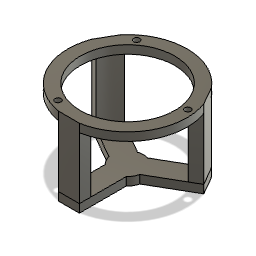
Speaker Mount Parts (Autodesk Fusion 360 design; units mm, degrees)
Autodesk Fusion 360 part; units mm, degrees
note: some values were not read from the file. Set by a fixed rule: which sketch regions a step uses; the direction of a hole.
sketch "Sketch1" plane through (0, 0, 0) normal (0, 1, 0) x (1, 0, 0)
  circle A0 centre (0, 0) radius 25.75
  line L0 (0, 0) -> (0, -25.75) construction
  line L1 (0, -30.75) -> (0, -25.75) construction
  line L2 (5.7222, -25.75) -> (-5.7222, -25.75)
  line L3 (-5.7222, -25.75) -> (-5.7222, -31.9923)
  line L4 (-5.7222, -31.9923) -> (5.7222, -31.9923)
  line L5 (5.7222, -31.9923) -> (5.7222, -25.75)
  circle A1 centre (0, 0) radius 32.5
  dimension "d1" = 51.5
  dimension "d62" = 11.4444
  dimension "d83" = 65
  constraint coincident A0.centre L0.start
  constraint coincident A0 L0.end
  constraint vertical L0
  constraint perpendicular L2 L3
  constraint parallel L2 L4
  constraint parallel L3 L5
  constraint perpendicular L1 L2
  constraint midpoint L0.end L2
  constraint concentric A0 A1
  constraint coincident L4.end A1
  constraint horizontal L2
  measures "d1" diameter of A0
  measures "d62" distance of L3.end L4.end
  measures "d83" diameter of A1
extrude "Extrude1" add sketch "Sketch1" along normal mid plane 4.5 makes body 1
extrude "Extrude6" cut sketch "Sketch1" along normal up to surface (2.25 mm away) and the other way up to surface (2.25 mm away) contours L4 A1 bodies 1
pattern_circular "C-Pattern2" count 3 over 360 about axis through (0, 1.75, 0) along (0, 1, 0) of "Extrude6"
ref_plane "WorkPlane1" through (0, 2.25, 0) normal (0, 1, 0) x (1, 0, 0)
sketch "Sketch10" plane through (0, -2.25, 0) normal (0, -1, 0) x (1, 0, 0)
  line L0 (-30.5672, -11.0406) -> (-24.845, -20.9517)
  arc A0 (-24.845, -20.9517) -> (24.845, -20.9517) centre (0, 0) ccw
  line L1 (24.845, -20.9517) -> (30.5672, -11.0406)
  arc A1 (30.5672, -11.0406) -> (5.7222, 31.9923) centre (0, 0) ccw
  line L2 (5.7222, 31.9923) -> (-5.7222, 31.9923)
  arc A2 (-5.7222, 31.9923) -> (-30.5672, -11.0406) centre (0, 0) ccw
  circle A3 centre (0, 0) radius 25.75
  line L3 (-5.7222, 31.9923) -> (-5.7222, 25.7468)
  line L4 (5.7222, 31.9923) -> (5.7222, 25.7468)
  line L5 (-24.845, -20.9517) -> (-19.4363, -17.829)
  line L6 (-30.5672, -11.0406) -> (-25.1585, -7.9178)
  line L7 (-30.5672, -11.0406) -> (-24.845, -20.9517)
  line L8 (30.5672, -11.0406) -> (25.1585, -7.9178)
  line L9 (24.845, -20.9517) -> (19.4363, -17.829)
  line L10 (24.845, -20.9517) -> (30.5672, -11.0406)
  circle A4 centre (0, 0) radius 26.375
  dimension "d90" = 360
  dimension "d91" = 52.75
  constraint coincident L2.end A2.start
  constraint perpendicular L2 L3
  constraint coincident A1.end L2.start
  constraint perpendicular L2 L4
  constraint concentric A0 A4
  constraint coincident L4.end A4
  constraint coincident L3.end A4
  measures "d91" diameter of A4
extrude "Extrude2" add sketch "Sketch10" along normal blind 33.5 contours L0 L5 L6 L7 A4 | L2 L3 L4 A4 | L1 L8 L9 L10 A4 bodies 1
sketch "Sketch3" plane through (0, -35.75, 0) normal (0, 1, 0) x (1, 0, 0)
  line L0 (0, -1.75) -> (0, -22.5)
  line L1 (-5.7222, -31.9923) -> (-5.7222, -6.3976)
  line L2 (5.7222, -31.9923) -> (5.7222, -6.3976)
  circle A0 centre (0, 0) radius 32.5
  line L3 (24.845, 20.9517) -> (2.6794, 8.1544)
  line L4 (30.5672, 11.0406) -> (8.4016, -1.7568)
  line L5 (-30.5672, 11.0406) -> (-8.4016, -1.7568)
  line L6 (-24.845, 20.9517) -> (-2.6794, 8.1544)
  circle A1 centre (0, 0) radius 8.5833
  line L7 (30.5672, 11.0406) -> (24.845, 20.9517)
  line L8 (24.845, 20.9517) -> (24.3966, 21.7285)
  line L9 (24.3966, 21.7285) -> (30.6869, 10.8333)
  line L10 (30.6869, 10.8333) -> (30.5672, 11.0406)
  line L11 (-24.7254, 21.159) -> (-24.845, 20.9517)
  line L12 (-31.0157, 10.2638) -> (-24.7254, 21.159)
  line L13 (-30.5672, 11.0406) -> (-31.0157, 10.2638)
  line L14 (-5.9616, -31.9923) -> (-5.7222, -31.9923)
  line L15 (6.6191, -31.9923) -> (-5.9616, -31.9923)
  line L16 (5.7222, -31.9923) -> (6.6191, -31.9923)
  arc A2 (24.8108, 6.8911) -> (18.3733, 18.0412) centre (0, 0) ccw
  line L17 (-25.1585, 7.9178) -> (-30.5672, 11.0406)
  line L18 (-30.5672, 11.0406) -> (-24.845, 20.9517)
  line L19 (-24.845, 20.9517) -> (-19.4363, 17.829)
  line L20 (27.7061, 15.9961) -> (22.3002, 12.875) construction
  arc A3 (-19.4363, 17.829) -> (-25.1585, 7.9178) centre (0, 0) ccw
  point P0 (25.0031, 14.4356)
  point P1 (-25.0031, 14.4356)
  point P2 (0, -28.8711)
  dimension "d21" = 5.7222
  dimension "d22" = 65
  dimension "d24" = 360
  dimension "d26" = 17.1667
  dimension "d44" = 360
  dimension "d55" = 360
  constraint vertical L1
  constraint symmetric L2.start L1.start L0
  constraint symmetric L2.end L1.end L0
  constraint coincident A0.centre A1.centre
  constraint concentric A0 A1
  constraint coincident L1.end A1
  constraint coincident L2.end A1
  constraint coincident L1.start A0
  constraint parallel L8 L10
  constraint collinear L7 L9
  constraint midpoint L7 L20.start
  constraint midpoint A2 L20.end
  constraint midpoint P0 L20
  measures "d21" distance of L0 L1
  measures "d22" diameter of A0
  measures "d26" diameter of A1
extrude "Extrude3" add sketch "Sketch3" against normal blind 4.5 separate body contours L1 L2 A1 L15 | A1 | L5 L6 L12 L17 L18 L19 A3 | L5 L6 A1 A3 | L3 L4 L7 L9 A2 | L3 L4 A1 A2 makes body 2
hole "Hole1" at (25.0031, -35.75, -14.4356) at (-25.0031, -35.75, -14.4356) at (0, -35.75, 28.8711) direction (0, -1, 0) diameter 3.3 end up to surface (4.5 mm away) bodies 2
hole "Hole5" at (-25.0031, -35.75, -14.4356) at (0, -35.75, 28.8711) at (25.0031, -35.75, -14.4356) direction (0, 1, 0) diameter 3.3 depth 7 tip angle 118 bodies 1
sketch "Sketch9" plane through (0, 2.25, 0) normal (0, 1, 0) x (1, 0, 0)
  arc A0 (-30.5672, 11.0406) -> (-5.7222, -31.9923) centre (0, 0) ccw
  arc A1 (5.7222, -6.3976) -> (8.4016, -1.7568) centre (0, 0) ccw
  line L0 (5.7222, -31.9923) -> (5.7222, -6.3976)
  line L1 (-5.7222, -31.9923) -> (5.7222, -31.9923)
  line L2 (-5.7222, -6.3976) -> (-5.7222, -31.9923)
  arc A2 (-8.4016, -1.7568) -> (-5.7222, -6.3976) centre (0, 0) ccw
  line L3 (-30.5672, 11.0406) -> (-8.4016, -1.7568)
  line L4 (-24.845, 20.9517) -> (-30.5672, 11.0406)
  line L5 (-2.6794, 8.1544) -> (-24.845, 20.9517)
  arc A3 (2.6794, 8.1544) -> (-2.6794, 8.1544) centre (0, 0) ccw
  line L6 (24.845, 20.9517) -> (2.6794, 8.1544)
  line L7 (30.5672, 11.0406) -> (24.845, 20.9517)
  line L8 (8.4016, -1.7568) -> (30.5672, 11.0406)
  line L9 (0, 0) -> (-10.9205, -27.0002) construction
  line L10 (-24.845, 20.9517) -> (-30.5672, 11.0406)
  line L11 (-5.7222, -31.9923) -> (5.7222, -31.9923)
  line L12 (30.5672, 11.0406) -> (24.845, 20.9517)
  circle A4 centre (0, 0) radius 25.75
  arc A5 (5.7222, -31.9923) -> (30.5672, 11.0406) centre (0, 0) ccw
  arc A6 (24.845, 20.9517) -> (-24.845, 20.9517) centre (0, 0) ccw
  circle A7 centre (-25.0031, 14.4356) radius 1.65
  circle A8 centre (25.0031, 14.4356) radius 1.65
  circle A9 centre (0, -28.8711) radius 1.65
  line L13 (-9.655, -23.8714) -> (-12.186, -30.1289) construction
  constraint coincident A0.centre A1.centre
  constraint coincident A4 L13.start
  constraint coincident A0 L13.end
  constraint parallel L9 L13
  constraint collinear L9 L13
  constraint coincident L9.end L13
  constraint midpoint L9.end L13
hole "Hole6" at (-10.9205, 2.25, 27.0002) direction (0, -1, 0) diameter 3.3 end up to surface (4.5 mm away) bodies 1
pattern_circular "C-Pattern4" count 3 over 360 about axis through (0, 1.75, 0) along (0, 1, 0) of "Hole6"
equation "d1 = InsideCircle"
equation "d3 = MiddleHeight"
equation "OutsideCircle = 65 mm"
equation "InsideCircle = 51.5 mm"
equation "ColumnWidth = InsideCircle / 4.5"
equation "d14 = Height - MiddleHeight + 8 mm"
equation "d21 = ColumnWidth / 2"
equation "d22 = OutsideCircle"
equation "Columns = 3"
equation "d26 = InsideCircle / 3"
equation "d28 = -MountHeights"
equation "MountHeights = 4.5 mm"
equation "InsertA = 3.5 mm"
equation "d56 = InsertA - 0.2 mm"
equation "d62 = ColumnWidth"
equation "SpeakerNonGrillHeight = 36 mm"
equation "MiddleHeight = 4.5 mm"
equation "d83 = OutsideCircle"
equation "Height = 30 mm"
equation "SpeakerD = 52.5 mm"
equation "d91 = SpeakerD + 0.25 mm"
equation "d93 = InsertA - 0.2 mm"
